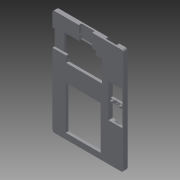
# Autodesk Inventor part: DisplayBottom2
Saved by Autodesk Inventor 2014 SP1 (Build 180222100, 222)
## iProperties
Created: 2014-03-24
Part Number: DisplayBottom2
Material: Generic
Document SubType Name: Modeling
Designer: patrigg
Density: 1 g/cm^3
Appearance: Default
Author: patrigg
Autodesk Inventor part; units mm, degrees
ref_plane "YZ Plane" through (0, 0, 0) normal (1, 0, 0) x (0, 1, 0)
ref_plane "XZ Plane" through (0, 0, 0) normal (0, 1, 0) x (-1, 0, 0)
ref_plane "XY Plane" through (0, 0, 0) normal (0, 0, 1) x (1, 0, 0)
sketch "Sketch2" plane through (0, 0, 0) normal (0, 1, 0) x (-1, 0, 0)
  line L0 (-33.5, -50) -> (33.5, -50)
  line L1 (33.5, -50) -> (33.5, 50)
  line L2 (33.5, 50) -> (-33.5, 50)
  line L3 (-33.5, 50) -> (-33.5, -50)
  line L4 (-33.5, -50) -> (33.5, 50) construction
  line L5 (33.5, -50) -> (-33.5, 50) construction
  point P0 (0, 0)
  dimension "d0" = 67
  dimension "d1" = 100
  constraints: 12 end point, 2 midpoint, 2 parallel, 1 horizontal, 1 perpendicular
  measures "d0" distance of L2.end L1.end
  measures "d1" distance of L1.end L0.end
extrude "Extrusion1" add sketch "Sketch2" along normal blind 4
sketch "Sketch3" plane through (0, 4, 0) normal (0, 1, 0) x (1, 0, 0)
  line L0 (33.5, 50) -> (-33.5, 50) projected
  line L1 (-23.5, -6.5) -> (14.5, -6.5)
  line L2 (14.5, -6.5) -> (14.5, 46)
  line L3 (14.5, 46) -> (-23.5, 46)
  line L4 (-23.5, 46) -> (-23.5, -6.5)
  line L5 (-23.5, -6.5) -> (14.5, 46) construction
  line L6 (14.5, -6.5) -> (-23.5, 46) construction
  line L7 (-33.5, 50) -> (-33.5, -50) projected
  point P0 (0, 0)
  point P1 (-4.5, 19.75)
  dimension "d4" = 38
  dimension "d5" = 52.5
  dimension "d6" = 4
  dimension "d111" = 10
  constraints: 12 end point, 2 midpoint, 2 parallel, 1 horizontal, 1 perpendicular
  measures "d4" distance of L3.end L2.end
  measures "d5" distance of L2.end L1.end
  measures "d6" distance between parallel lines of L0 L3
  measures "d111" distance between parallel lines of L4 L7
extrude "Extrusion2" cut sketch "Sketch3" against normal blind 1.5
sketch "Sketch4" plane through (0, 2.5, 0) normal (0, 1, 0) x (1, 0, 0)
  line L0 (14.5, -6.5) -> (-23.5, -6.5) projected
  line L1 (14.5, 46) -> (14.5, -6.5) projected
  line L2 (-23.5, 46) -> (14.5, 46) projected
  line L3 (-23.5, -6.5) -> (-23.5, 46) projected
  line L4 (-21, 44.5) -> (12, 44.5)
  line L5 (12, 44.5) -> (12, 3.5)
  line L6 (12, 3.5) -> (-21, 3.5)
  line L7 (-21, 3.5) -> (-21, 44.5)
  line L8 (-21, 44.5) -> (12, 3.5) construction
  line L9 (12, 44.5) -> (-21, 3.5) construction
  point P0 (0, 0)
  point P1 (-4.5, 24)
  dimension "d9" = 10
  dimension "d10" = 1.5
  dimension "d11" = 2.5
  dimension "d12" = 2.5
  constraints: 12 end point, 2 midpoint, 2 parallel, 1 horizontal, 1 perpendicular
  measures "d9" distance between parallel lines of L0 L6
  measures "d10" distance between parallel lines of L2 L4
  measures "d11" distance between parallel lines of L1 L5
  measures "d12" distance between parallel lines of L3 L7
extrude "Extrusion3" cut sketch "Sketch4" against normal blind 2.5 contours L4 L5 L6 L7
sketch "Sketch12" plane through (0, 4, 0) normal (0, 1, 0) x (1, 0, 0)
  line L0 (-24.5, -37) -> (13.5, -37)
  line L1 (13.5, -37) -> (13.5, -13)
  line L2 (13.5, -13) -> (-24.5, -13)
  line L3 (-24.5, -13) -> (-24.5, -37)
  line L4 (-24.5, -37) -> (13.5, -13) construction
  line L5 (13.5, -37) -> (-24.5, -13) construction
  line L6 (-23.5, -6.5) -> (-23.5, 46) projected
  line L7 (14.5, -6.5) -> (-23.5, -6.5) projected
  point P0 (0, 0)
  point P1 (-5.5, -25)
  point P2 (-5.5, -25)
  dimension "d58" = 38
  dimension "d59" = 24
  dimension "d112" = 1
  dimension "d154" = 6.5
  constraints: 12 end point, 3 midpoint, 2 parallel, 1 horizontal, 1 perpendicular
  measures "d58" distance of L2.end L1.end
  measures "d59" distance of L1.end L0.end
  measures "d112" distance between parallel lines of L3 L6
  measures "d154" distance between parallel lines of L7 L2
extrude "Extrusion10" cut sketch "Sketch12" against normal blind 4
sketch "Sketch18" plane through (13.5, 4, 13) normal (-1, 0, 0) x (0, 0, 1)
  line L0 (0, 0) -> (24, 0) projected
  line L1 (24, -4) -> (20, -4)
  line L2 (20, -4) -> (20, -1.8)
  line L3 (20, -1.8) -> (24, -1.8)
  line L4 (24, -1.8) -> (24, -4)
  point P0 (-13, -4)
  dimension "d88" = 4
  dimension "d89" = 1.8
  constraints: 8 end point, 2 parallel, 1 horizontal, 1 perpendicular
  measures "d88" distance of L2.end L3.end
  measures "d89" distance between parallel lines of L3 L0
extrude "Extrusion17" add sketch "Sketch18" along normal blind 6
sketch "Sketch20" plane through (-24.5, 4, 37) normal (1, 0, 0) x (0, 0, -1)
  line L0 (0, 0) -> (24, 0) projected
  line L1 (24, -4) -> (18, -4)
  line L2 (18, -4) -> (18, -1.8)
  line L3 (18, -1.8) -> (24, -1.8)
  line L4 (24, -1.8) -> (24, -4)
  point P0 (37, -4)
  dimension "d96" = 6
  dimension "d97" = 1.8
  constraints: 8 end point, 2 parallel, 1 horizontal, 1 perpendicular
  measures "d96" distance of L2.end L3.end
  measures "d97" distance between parallel lines of L3 L0
extrude "Extrusion19" add sketch "Sketch20" along normal blind 4
sketch "Sketch22" plane through (0, 0, 0) normal (0, -1, 0) x (1, 0, 0)
  line L0 (33.5, 50) -> (33.5, -50) projected
  line L1 (32.5, -14) -> (19.5, -14)
  line L2 (19.5, -14) -> (19.5, 18)
  line L3 (19.5, 18) -> (32.5, 18)
  line L4 (32.5, 18) -> (32.5, -14)
  line L5 (33.5, -50) -> (-33.5, -50) projected
  point P0 (0, 0)
  dimension "d102" = 1
  dimension "d103" = 13
  dimension "d110" = 32
  dimension "d155" = 36
  constraints: 8 end point, 2 parallel, 1 horizontal, 1 perpendicular
  measures "d102" distance between parallel lines of L4 L0
  measures "d103" distance between parallel lines of L2 L4
  measures "d110" distance between parallel lines of L3 L1
  measures "d155" distance between parallel lines of L5 L1
extrude "Extrusion21" cut sketch "Sketch22" against normal up to next
sketch "Sketch23" plane through (0, 4, 0) normal (0, 1, 0) x (1, 0, 0)
  line L0 (-24.5, -13) -> (13.5, -13) projected
  line L1 (14.5, 46) -> (14.5, -6.5) projected
  line L2 (14.5, -6.5) -> (-23.5, -6.5) projected
  line L3 (-23.5, -6.5) -> (-23.5, 46) projected
  line L4 (-21.5, -6.5) -> (-21.5, -13)
  line L5 (12.5, -6.5) -> (12.5, -13)
  point P0 (0, 0)
  dimension "d114" = 2
  dimension "d115" = 2
  constraints: 4 end point, 4 point on line, 2 perpendicular
  measures "d114" distance between parallel lines of L4 L3
  measures "d115" distance between parallel lines of L1 L5
extrude "Extrusion22" cut sketch "Sketch23" against normal up to surface (1.5 mm away)
sketch "Sketch24" plane through (32.5, 0, -14) normal (-1, 0, 0) x (0, 0, 1)
  line L0 (0, 0) -> (0, 4) projected
  line L1 (14.5, 2) -> (17.5, 2)
  line L2 (17.5, 2) -> (17.5, 4)
  line L3 (17.5, 4) -> (14.5, 4)
  line L4 (14.5, 4) -> (14.5, 2)
  line L5 (14.5, 2) -> (17.5, 4) construction
  line L6 (17.5, 2) -> (14.5, 4) construction
  line L7 (0, 4) -> (32, 4) projected
  point P0 (16, 3)
  dimension "d118" = 3
  dimension "d119" = 2
  dimension "d120" = 16
  constraints: 12 end point, 2 midpoint, 2 parallel, 1 collinear, 1 horizontal, 1 perpendicular
  measures "d118" distance of L3.end L2.end
  measures "d119" distance of L2.end L1.end
  measures "d120" distance from line of L0 point (16, 3)
extrude "Extrusion23" add sketch "Sketch24" along normal up to next
sketch "Sketch25" plane through (32.5, 2, 0.5) normal (0, -1, 0) x (1, 0, 0)
  line L0 (-8, 1) -> (-5, 1)
  line L1 (-5, 1) -> (-5, 3)
  line L2 (-5, 3) -> (-8, 3)
  line L3 (-8, 3) -> (-8, 1)
  line L4 (-8, 1) -> (-5, 3) construction
  line L5 (-5, 1) -> (-8, 3) construction
  line L6 (0, 3) -> (-13, 3) projected
  point P0 (32.5, 26.5)
  point P1 (-6.5, 2)
  point P2 (-6.5, 2)
  point P3 (-6.5, 0)
  point P4 (-6.5, 2)
  point P5 (-6.5, 3)
  dimension "d123" = 3
  dimension "d124" = 2
  constraints: 12 end point, 5 midpoint, 2 parallel, 2 vertical alignment, 1 collinear, 1 horizontal, 1 perpendicular
  measures "d123" distance of L2.end L1.end
  measures "d124" distance of L1.end L0.end
extrude "Extrusion24" cut sketch "Sketch25" against normal blind 0.5
fillet "Fillet6" radius 1 1 edges at (26, 2.5, 3.5)
sketch "Sketch26" plane through (32.5, 2, 0.5) normal (0, -1, 0) x (1, 0, 0)
  line L0 (0, 3) -> (0, 0)
  circle A0 centre (-10.625, 1.5) radius 1.25
  circle A1 centre (-2.375, 1.5) radius 1.25
  line L1 (0, 3) -> (-13, 3) projected
  line L2 (-13, -14.5) -> (-13, 17.5) projected
  point P0 (32.5, 26.5)
  point P1 (-6.5, 1.5)
  point P2 (0, 1.5)
  point P3 (-6.5, 0)
  point P4 (-6.5, 3)
  point P5 (-13, 1.5)
  dimension "d128" = 2.5
  dimension "d129" = 2.5
  dimension "d130" = 4.125
  dimension "d131" = 8.25
  constraints: 4 horizontal alignment, 3 midpoint, 2 centre point, 2 end point, 2 vertical alignment
  measures "d128" diameter of A0
  measures "d129" diameter of A1
  measures "d130" distance of point (-6.5, 1.5) A0.centre
  measures "d131" distance of A1.centre A0.centre
extrude "Extrusion25" add sketch "Sketch26" along normal blind 2
chamfer "Chamfer3" distance 0.5 angle 45 2 edges at (28.875, 0, 2) (20.625, 0, 2)
sketch "Sketch27" plane through (0, 4, 0) normal (0, 1, 0) x (1, 0, 0)
  line L0 (-33.5, -50) -> (33.5, -50) projected
  line L1 (32.5, -18) -> (19.5, -18) projected
  line L2 (19.5, 14) -> (32.5, 14) projected
  line L3 (15.25, -50) -> (25.75, -50)
  line L4 (25.75, -50) -> (25.75, -32)
  line L5 (25.75, -32) -> (15.25, -32)
  line L6 (15.25, -32) -> (15.25, -50)
  line L7 (15.25, -50) -> (25.75, -32) construction
  line L8 (25.75, -50) -> (15.25, -32) construction
  line L9 (19.5, -18) -> (19.5, 14) projected
  line L10 (15.25, -42) -> (15.5, -42)
  line L11 (15.5, -42) -> (15.5, -32)
  line L12 (25.75, -42) -> (25.5, -42)
  line L13 (25.5, -42) -> (25.5, -32)
  point P0 (0, 0)
  point P1 (26, 14)
  point P2 (20.5, -41)
  point P3 (20.5, -41)
  point P4 (26, -18)
  dimension "d138" = 10.5
  dimension "d139" = 18
  dimension "d148" = 0.25
  dimension "d149" = 0.25
  dimension "d150" = 8
  dimension "d168" = 13
  constraints: 20 end point, 5 midpoint, 5 perpendicular, 4 point on line, 2 collinear, 2 parallel, 1 horizontal
  measures "d138" distance of L5.end L4.end
  measures "d139" distance of L4.end L3.end
  measures "d148" distance between parallel lines of L11 L6
  measures "d149" distance between parallel lines of L4 L13
  measures "d150" distance from line of L0 L10.end
  measures "d168" horizontal distance of L0.end point (20.5, -41)
extrude "Extrusion26" cut sketch "Sketch27" against normal blind 2.5 contours L6 L10 L11 L5 L13 L12 L4 L0
sketch "Sketch29" plane through (0, 0, 0) normal (0, -1, 0) x (1, 0, 0)
  line L0 (-24.5, 19) -> (-24.5, 37) projected
  line L1 (-24.5, 37) -> (7.5, 37) projected
  line L2 (-33.5, -50) -> (-33.5, 50) projected
  line L3 (-33.5, 50) -> (33.5, 50) projected
  line L4 (-24.5, 19) -> (-33.5, 19)
  line L5 (-24.5, 35.5) -> (-33.5, 35.5)
  point P0 (0, 0)
  dimension "d151" = 1.5
  constraints: 4 end point, 3 point on line, 1 parallel, 1 perpendicular
  measures "d151" distance between parallel lines of L1 L5
extrude "Extrusion28" cut sketch "Sketch29" against normal blind 2
sketch "Sketch30" plane through (0, 0, 0) normal (0, -1, 0) x (1, 0, 0)
  line L0 (-33.5, 50) -> (33.5, 50) projected
  line L1 (-8.5, 42) -> (4, 42)
  line L2 (4, 42) -> (4, 50)
  line L3 (4, 50) -> (-8.5, 50)
  line L4 (-8.5, 50) -> (-8.5, 42)
  line L5 (-8.5, 42) -> (4, 50) construction
  line L6 (4, 42) -> (-8.5, 50) construction
  line L7 (3.75, 37) -> (-8.25, 37)
  line L8 (-8.25, 37) -> (-8.25, 42)
  line L9 (-8.25, 42) -> (3.75, 42)
  line L10 (3.75, 42) -> (3.75, 37)
  line L11 (3.75, 37) -> (-8.25, 42) construction
  line L12 (-8.25, 37) -> (3.75, 42) construction
  line L13 (-24.5, 37) -> (7.5, 37) projected
  point P0 (0, 0)
  point P1 (-2.25, 46)
  point P2 (-2.25, 39.5)
  point P3 (-2.25, 39.5)
  point P4 (-2.25, 46)
  dimension "d156" = 12.5
  dimension "d157" = 8
  dimension "d158" = 16
  dimension "d162" = 12
  constraints: 24 end point, 6 midpoint, 4 parallel, 2 collinear, 2 horizontal, 2 perpendicular, 1 point on line, 1 vertical alignment
  measures "d156" distance of L3.end L2.end
  measures "d157" distance of L2.end L1.end
  measures "d158" distance from line of L4 L13.start
  measures "d162" distance between parallel lines of L8 L10
extrude "Extrusion29" cut sketch "Sketch30" against normal blind 2.5
sketch "Sketch32" plane through (0, 2.5, 0) normal (0, -1, 0) x (1, 0, 0)
  line L0 (-8.25, 37) -> (-8.25, 42) projected
  line L1 (3.75, 37) -> (-8.25, 37) projected
  line L2 (3.75, 42) -> (3.75, 37) projected
  line L3 (-8.25, 42) -> (-8.5, 42) projected
  line L4 (-8.25, 38) -> (3.75, 38)
  point P0 (0, 0)
  dimension "d183" = 1
  constraints: 2 end point, 2 point on line, 1 parallel
  measures "d183" distance between parallel lines of L1 L4
extrude "Extrusion31" add sketch "Sketch32" along normal blind 0.5
sketch "Sketch33" plane through (0, 4, 0) normal (0, 1, 0) x (1, 0, 0)
  line L0 (27.25, 14) -> (27.25, 21.5)
  line L1 (27.25, 21.5) -> (15.5, 21.5)
  line L2 (15.5, 21.5) -> (15.5, -24.5)
  line L3 (24.75, 14) -> (24.75, 19)
  line L4 (24.75, 19) -> (18, 19)
  line L5 (18, 19) -> (18, -19.9289)
  line L6 (18, -19.9289) -> (23, -24.9289)
  line L7 (23, -24.9289) -> (23, -32)
  line L8 (15.5, -24.5) -> (18, -27)
  line L9 (18, -27) -> (18, -32)
  line L10 (19.5, 14) -> (32.5, 14) projected
  line L11 (18, -32) -> (23, -32)
  line L12 (24.75, 14) -> (27.25, 14)
  line L13 (15.5, -32) -> (25.5, -32) projected
  line L14 (13.5, -13) -> (13.5, -37) projected
  point P0 (0, 0)
  point P1 (26, 14)
  point P2 (20.5, -32)
  point P3 (20.5, -32)
  point P4 (26, 14)
  point P5 (20.5, -32)
  dimension "d198" = 2.5
  dimension "d199" = 2.5
  dimension "d200" = 2.5
  dimension "d201" = 5
  dimension "d202" = 5
  dimension "d203" = 135
  dimension "d204" = 135
  dimension "d205" = 2.5
  dimension "d206" = 1.25
  dimension "d207" = 2
  dimension "d208" = 5
  dimension "d209" = 5
  constraints: 24 end point, 3 horizontal alignment, 3 midpoint, 3 perpendicular, 2 coincident, 2 parallel
  measures "d198" distance between parallel lines of L5 L2
  measures "d199" distance between parallel lines of L1 L4
  measures "d200" distance between parallel lines of L0 L3
  measures "d201" distance between parallel lines of L7 L9
  measures "d202" distance from line of L5.end L8
  measures "d203" angle of L5 L6
  measures "d204" angle of L2 L8
  measures "d205" distance from line of L7 point (20.5, -32)
  measures "d206" distance of L0.start point (26, 14)
  measures "d207" distance between parallel lines of L14 L2
  measures "d208" distance of L9.end L8.end
  measures "d209" distance between parallel lines of L10 L4
extrude "Extrusion32" cut sketch "Sketch33" against normal up to surface (2.5 mm away)
chamfer "Chamfer6" distance 2 angle 45 2 edges at (24.75, 2.75, -14) (27.25, 2.75, -14)
fillet "Fillet9" radius 2 13 edges at (22.75, 2.75, -14) (27.25, 2.75, -16) (29.25, 2.75, -14) (27.25, 2.75, -21.5) (15.5, 2.75, -21.5) (18, 2.75, 19.9289) (23, 2.75, 24.9289) (23, 2.75, 32) (18, 2.75, 32) (18, 2.75, 27) (15.5, 2.75, 24.5) (24.75, 2.75, -16) (24.75, 2.75, -19)
fillet "Fillet9" radius 2 1 edges at (18, 2.75, -19)
fillet "Fillet10" radius 2 4 edges at (33.5, 2, 50) (-33.5, 2, 50) (33.5, 2, -50) (-33.5, 2, -50)
body "Solid1"
